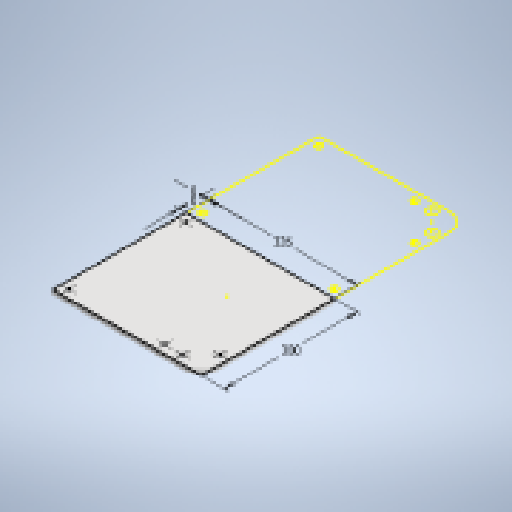
# Autodesk Inventor part: Right bottom plate
Saved by Autodesk Inventor 2024 (Build 280153000, 153)
## iProperties
Created: 2024-03-26
Part Number: Right bottom plate
Material: Generic
Document SubType Name: Modeling
Designer: jens1
Density: 1 g/cm^3
Appearance: Default
Author: jens1
Autodesk Inventor part; units mm, degrees
ref_plane "YZ Plane" through (0, 0, 0) normal (1, 0, 0) x (0, 1, 0)
ref_plane "XZ Plane" through (0, 0, 0) normal (0, 1, 0) x (-1, 0, 0)
ref_plane "XY Plane" through (0, 0, 0) normal (0, 0, 1) x (1, 0, 0)
sketch "Sketch1" plane through (0, 0, 0) normal (0, 1, 0) x (-1, 0, 0)
  line L0 (211.3942, 181.6544) -> (-123.6058, 181.6544)
  line L1 (-123.6058, 181.6544) -> (-123.6058, -118.3456)
  line L2 (-123.6058, -118.3456) -> (211.3942, -118.3456)
  line L3 (211.3942, -118.3456) -> (211.3942, 181.6544)
  arc A0 (-123.6058, -378.3456) -> (-83.6058, -418.3456) centre (-83.6058, -378.3456) ccw projected
  line L4 (-83.6058, -418.3456) -> (211.3942, -418.3456) projected
  line L5 (211.3942, -418.3456) -> (211.3942, -118.3456) projected
  line L6 (211.3942, -118.3456) -> (-123.6058, -118.3456) projected
  line L7 (-123.6058, -118.3456) -> (-123.6058, -378.3456) projected
  circle A1 centre (-104.7558, -357.4956) radius 11.75 projected
  circle A2 centre (-62.7558, -399.4956) radius 11.75 projected
  circle A3 centre (-104.7558, -137.1956) radius 7.85 projected
  circle A4 centre (-104.7558, -317.8956) radius 7.85 projected
  circle A5 centre (-23.1558, -399.4956) radius 7.85 projected
  circle A6 centre (192.5442, -399.4956) radius 7.85 projected
  circle A7 centre (192.5442, -137.1956) radius 7.85 projected
  point P0 (0, 0)
  point P1 (-104.7558, 120.8044)
  point P2 (-62.7558, 162.8044)
  point P3 (-23.1558, 162.8044)
  point P4 (192.5442, 162.8044)
  point P5 (192.5442, -99.4956)
  point P6 (192.5442, 162.8044)
  point P7 (-23.1558, 162.8044)
  point P8 (-62.7558, 162.8044)
  point P9 (-104.7558, 120.8044)
  point P10 (192.5442, -99.4956)
  dimension "d0" = 335
  dimension "d1" = 300
  dimension "d2" = 0
  dimension "d3" = 0
  constraints: 8 end point, 5 coincident, 5 symmetric about line, 2 parallel, 1 horizontal, 1 perpendicular
  measures "d0" distance of L2.end L1.end
  measures "d1" distance of L1.end L0.end
  measures "d2" distance between parallel lines of L6 L2
  measures "d3" distance between parallel lines of L5 L3
extrude "Extrusion1" add sketch "Sketch1" against normal blind 10.5 contours L3 L2 L1 L0
hole "Hole1" at (-192.5442, 0, 162.8044) at (23.1558, 0, 162.8044) at (-192.5442, 0, -99.4956) direction (0, -1, 0) diameter 8 end through all countersink diameter 15.7 countersink angle 90
hole "Hole2" at (62.7558, 0, 162.8044) at (104.7558, 0, 120.8044) direction (0, -1, 0) diameter 12 end through all countersink diameter 23.5 countersink angle 90
fillet "Fillet1" radius 40 1 edges at (123.6058, -5.25, 181.6544)
body "Solid1"
